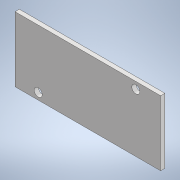
# Autodesk Inventor part: XL4015
Saved by Autodesk Inventor 2022 (Build 260153070, 153G)
## iProperties
Created: 2022-02-15
Part Number: XL4015
Material: Generic
Document SubType Name: Modeling
Designer: a laptop
Density: 1 g/cm^3
Appearance: Default
Author: a laptop
Autodesk Inventor part; units mm, degrees
ref_plane "YZ Plane" through (0, 0, 0) normal (1, 0, 0) x (0, 1, 0)
ref_plane "XZ Plane" through (0, 0, 0) normal (0, 1, 0) x (-1, 0, 0)
ref_plane "XY Plane" through (0, 0, 0) normal (0, 0, 1) x (1, 0, 0)
sketch "Sketch1" plane through (0, 0, 0) normal (0, 0, 1) x (1, 0, 0)
  line L0 (0, 24.2) -> (54.2, 24.2)
  line L1 (54.2, 24.2) -> (54.2, 0)
  line L2 (54.2, 0) -> (0, 0)
  line L3 (0, 0) -> (0, 24.2)
  circle A0 centre (44.95, 21.7) radius 1.5
  circle A1 centre (8.6, 2.5) radius 1.5
  dimension "d0" = 54.2
  dimension "d1" = 24.2
  dimension "d2" = 3
  dimension "d3" = 2.5
  dimension "d4" = 9.25
  dimension "d5" = 2.5
  dimension "d6" = 8.6
  constraints: 8 end point, 2 centre point, 2 parallel, 1 coincident, 1 equal radius, 1 horizontal, 1 perpendicular
  measures "d0" distance of L0.start L0.end
  measures "d1" distance of L0.end L1.end
  measures "d2" diameter of A0
  measures "d3" distance from line of L0 A0.centre
  measures "d4" distance from line of L1 A0.centre
  measures "d5" distance from line of L2 A1.centre
  measures "d6" distance from line of L3 A1.centre
extrude "Extrusion1" add sketch "Sketch1" along normal blind 1.6
body "Solid1"
